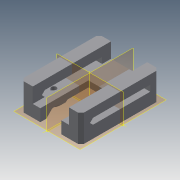
# Autodesk Inventor part: HbSensorHolder02
Saved by Autodesk Inventor 2015 SP1 (Build 190203100, 203)
## iProperties
Created: 2016-01-24
Part Number: HbSensorHolder02
Material: Generic
Document SubType Name: Modeling
Designer: Yamaura
Density: 1 g/cm^3
Appearance: Default
Author: Yamaura
Autodesk Inventor part; units mm, degrees
sketch "スケッチ1" plane through (0, 0, 0) normal (0, 1, 0) x (-1, 0, 0)
  line L0 (10, -13) -> (-10, -13)
  line L1 (-10, -13) -> (-10, 13)
  line L2 (-10, 13) -> (10, 13)
  line L3 (10, 13) -> (10, -13)
  line L4 (10, -13) -> (-10, 13) construction
  line L5 (-10, -13) -> (10, 13) construction
  point P0 (0, 0)
  dimension "d0" = 20
  dimension "d1" = 26
  constraints: 12 end point, 2 midpoint, 2 parallel, 1 horizontal, 1 perpendicular
  measures "d0" distance of L1.end L2.end
  measures "d1" distance of L0.end L1.end
extrude "押し出し1" add sketch "スケッチ1" along normal blind 4
shell "シェル1" thickness 2 removed faces 1 at (-3.3333, 0, -4.3333)
sketch "スケッチ2" plane through (0, 0, 0) normal (0, 1, 0) x (-1, 0, 0)
  line L0 (3.5, 13) -> (-3.5, 13)
  line L1 (-3.5, 13) -> (-3.5, -3)
  line L2 (-3.5, -3) -> (3.5, -3)
  line L3 (3.5, -3) -> (3.5, 13)
  point P0 (0, 0)
  dimension "d5" = 7
  dimension "d6" = 16
  dimension "d7" = 3
  dimension "d8" = 3.5
  constraints: 8 end point, 2 parallel, 1 horizontal, 1 perpendicular
  measures "d5" distance of L2.end L1.end
  measures "d6" distance of L1.end L0.end
  measures "d7" distance from line of L2 point (0, 0)
  measures "d8" distance from line of L3 point (0, 0)
extrude "押し出し2" cut sketch "スケッチ2" along normal blind 4
sketch "スケッチ3" plane through (0, 0, 0) normal (0, 1, 0) x (-1, 0, 0)
  circle A0 centre (7, 5) radius 2
  circle A1 centre (-7, -5) radius 2
  point P0 (0, 0)
  dimension "d11" = 4
  dimension "d12" = 4
  dimension "d13" = 5
  dimension "d14" = 5
  dimension "d15" = 7
  dimension "d16" = 7
  constraints: 2 centre point
  measures "d11" diameter of A0
  measures "d12" diameter of A1
  measures "d13" vertical distance of A0.centre point (0, 0)
  measures "d14" vertical distance of A1.centre point (0, 0)
  measures "d15" horizontal distance of point (0, 0) A1.centre
  measures "d16" horizontal distance of point (0, 0) A0.centre
extrude "押し出し3" add sketch "スケッチ3" along normal blind 4
sketch "スケッチ4" plane through (0, 0, 0) normal (0, 1, 0) x (-1, 0, 0)
  line L0 (8, 6.7321) -> (8, 11) projected
  line L1 (8, 11) -> (3.5, 11) projected
  line L2 (3.5, 11) -> (3.5, 13) projected
  line L3 (3.5, 13) -> (10, 13) projected
  line L4 (10, 13) -> (10, -13) projected
  line L5 (10, -13) -> (-10, -13) projected
  line L6 (-10, -13) -> (-10, 13) projected
  line L7 (-10, 13) -> (-3.5, 13) projected
  line L8 (-3.5, 13) -> (-3.5, 11) projected
  line L9 (-3.5, 11) -> (-8, 11) projected
  line L10 (-8, 11) -> (-8, -3.2679) projected
  arc A0 (-8, -6.7321) -> (-8, -3.2679) centre (-7, -5) ccw projected
  line L11 (-8, -6.7321) -> (-8, -11) projected
  line L12 (-8, -11) -> (8, -11) projected
  line L13 (8, -11) -> (8, 3.2679) projected
  arc A1 (8, 6.7321) -> (8, 3.2679) centre (7, 5) ccw projected
  circle A2 centre (7, 5) radius 0.85
  circle A3 centre (-7, -5) radius 0.85
  point P0 (0, 0)
  dimension "d19" = 1.7
  dimension "d20" = 1.7
  dimension "d55" = 7
  dimension "d56" = 5
  constraints: 2 centre point, 2 coincident
  measures "d19" diameter of A2
  measures "d20" diameter of A3
  measures "d55" horizontal distance of A1.centre point (0, 0)
  measures "d56" vertical distance of A1.centre point (0, 0)
extrude "押し出し4" cut sketch "スケッチ4" along normal blind 4 contours A2 | A3
sketch "スケッチ5" plane through (10, 0, 13) normal (1, 0, 0) x (0, 0, -1)
  line L0 (2, 2) -> (16.2679, 2) projected
  line L1 (26, 0) -> (0, 0) projected
  line L2 (26, 0) -> (26, 4) projected
  line L3 (0, 4) -> (26, 4) projected
  line L4 (0, 0) -> (0, 4) projected
  line L5 (0, 4) -> (26, 4)
  line L6 (26, 4) -> (26, 9)
  line L7 (26, 9) -> (0, 9)
  line L8 (0, 9) -> (0, 4)
  line L9 (3, 4) -> (23, 4)
  line L10 (23, 4) -> (23, 6)
  line L11 (23, 6) -> (3, 6)
  line L12 (3, 6) -> (3, 4)
  point P0 (13, 0)
  dimension "d23" = 26
  dimension "d24" = 5
  dimension "d25" = 3
  dimension "d26" = 3
  dimension "d27" = 3
  constraints: 16 end point, 4 parallel, 2 horizontal, 2 perpendicular, 1 point on line
  measures "d23" distance of L7.end L6.end
  measures "d24" distance of L6.end L5.end
  measures "d25" distance between parallel lines of L12 L8
  measures "d26" distance between parallel lines of L6 L10
  measures "d27" distance between parallel lines of L11 L7
extrude "押し出し5" add sketch "スケッチ5" against normal blind 4 contours L3 L10 L11 L12 L8 L7 L6
mirror "ミラー1" about plane through (0, 0, 0) normal (1, 0, 0) of "押し出し5"
chamfer "面取り1" distance 1 angle 45 4 edges at (10, 4.5, 13) (10, 4.5, -13) (-10, 4.5, -13) (-10, 4.5, 13)
sketch "スケッチ6" plane through (0, 0, 0) normal (0, -1, 0) x (1, 0, 0)
  circle A0 centre (7, -5) radius 0.85 projected
  circle A1 centre (-7, 5) radius 0.85 projected
  line L0 (-10, 12) -> (-9, 13) projected
  line L1 (-10, 12) -> (-10, -12) projected
  line L2 (-9, -13) -> (-10, -12) projected
  line L3 (-9, -13) -> (9, -13) projected
  line L4 (10, -12) -> (9, -13) projected
  line L5 (10, -12) -> (10, 12) projected
  line L6 (9, 13) -> (10, 12) projected
  line L7 (9, 13) -> (3.5, 13) projected
  line L8 (3.5, 13) -> (3.5, 11) projected
  line L9 (3.5, 11) -> (8, 11) projected
  line L10 (8, 11) -> (8, -3.2679) projected
  arc A2 (5, -5) -> (8, -6.7321) centre (7, -5) ccw
  line L11 (8, -6.7321) -> (8, -11) projected
  line L12 (8, -11) -> (-8, -11) projected
  line L13 (-8, -11) -> (-8, 3.2679) projected
  arc A3 (-8, 3.2679) -> (-5, 5) centre (-7, 5) ccw
  line L14 (-8, 6.7321) -> (-8, 11) projected
  line L15 (-8, 11) -> (-3.5, 11) projected
  line L16 (-3.5, 11) -> (-3.5, 13) projected
  line L17 (-3.5, 13) -> (-9, 13) projected
  line L18 (-5, 5) -> (-5, 1)
  line L19 (-5, 1) -> (-8, 1)
  line L20 (-8, 1) -> (-8, 3.2679)
  line L21 (8, -6.7321) -> (8, -9)
  line L22 (8, -9) -> (5, -9)
  line L23 (5, -9) -> (5, -5)
  point P0 (0, 0)
  dimension "d34" = 1
  dimension "d35" = 2
  dimension "d36" = 4
  dimension "d37" = 4
  constraints: 12 end point, 6 point on circle, 5 centre point, 2 parallel
  measures "d34" distance from line of L20 A1.centre
  measures "d35" distance from line of L18 A1.centre
  measures "d36" distance from line of L19 A1.centre
  measures "d37" distance from line of L22 A0.centre
extrude "押し出し6" add sketch "スケッチ6" against normal up to surface (2 mm away) contours A2 L11 L22 L23 | L13 A3 L18 L19
chamfer "面取り2" distance 2 angle 45 2 edges at (-6.5, 0, 1) (6.5, 0, -9)
chamfer "面取り3" distance 1 angle 45 4 edges at (8, 4, 10) (8, 6, 10) (-8, 4, 10) (-8, 6, 10)
chamfer "面取り4" distance 2 angle 45 2 edges at (-5.75, 2, 11) (5.75, 2, 11)
sketch "スケッチ7" plane through (0, 0, 0) normal (0, -1, 0) x (1, 0, 0)
  line L0 (-10, 9) -> (-6, 9) projected
  line L1 (-10, 9) -> (-10, -10) projected
  line L2 (-10, -10) -> (-6, -10) projected
  line L3 (-6, -10) -> (-6, 9) projected
  circle A0 centre (-7, 5) radius 0.85 projected
  circle A1 centre (7, -5) radius 0.85 projected
  line L4 (-7, 5) -> (-6.399, 5.601)
  line L5 (-6.399, 5.601) -> (-7, 6.2021)
  line L6 (-7, 6.2021) -> (-7.601, 5.601)
  line L7 (-7.601, 5.601) -> (-7, 5)
  line L8 (7, -5) -> (7.601, -4.399)
  line L9 (7.601, -4.399) -> (7, -3.7979)
  line L10 (7, -3.7979) -> (6.399, -4.399)
  line L11 (6.399, -4.399) -> (7, -5)
  point P0 (0, 0)
  dimension "d49" = 0.85
  dimension "d50" = 0.85
  dimension "d51" = 0.85
  dimension "d52" = 0.85
  constraints: 16 end point, 4 parallel, 2 perpendicular
  measures "d49" distance of L6.end L5.end
  measures "d50" distance of L5.end L4.end
  measures "d51" distance of L10.end L9.end
  measures "d52" distance of L9.end L8.end
extrude "押し出し7" cut sketch "スケッチ7" against normal blind 4 contours L4 L7 A0 | A0 L6 L5 | L8 L11 A1 | A1 L10 L9 picked at (-7, 5.5631) picked at (7, -4.4369)
